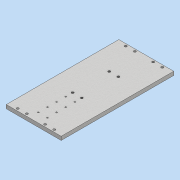
# Autodesk Inventor part: Wspornik pionowy osi Z
Saved by Autodesk Inventor 2018 (Build 220112000, 112)
## iProperties
Created: 2019-01-27
Part Number: Wspornik pionowy osi Z
Material: Ogólny
Document SubType Name: Modeling
Designer: Dawid
Density: 1 g/cm^3
Appearance: Aluminium odlewane
Author: Dawid
Autodesk Inventor part; units mm, degrees
ref_plane "YZ Plane" through (0, 0, 0) normal (1, 0, 0) x (0, 1, 0)
ref_plane "XZ Plane" through (0, 0, 0) normal (0, 1, 0) x (-1, 0, 0)
ref_plane "XY Plane" through (0, 0, 0) normal (0, 0, 1) x (1, 0, 0)
sketch "Szkic1" plane through (0, 0, 0) normal (0, 0, 1) x (1, 0, 0)
  line L0 (-50, -65) -> (50, -65)
  line L1 (50, -65) -> (50, 65)
  line L2 (50, 65) -> (-50, 65)
  line L3 (-50, 65) -> (-50, -65)
  line L4 (-50, -65) -> (50, 65) construction
  line L5 (50, -65) -> (-50, 65) construction
  point P0 (0, 0)
  dimension "d0" = 100
  dimension "d1" = 130
  constraints: 12 end point, 2 midpoint, 2 parallel, 1 horizontal, 1 perpendicular
  measures "d0" distance of L2.end L1.end
  measures "d1" distance of L1.end L0.end
extrude "Wyciągnięcie proste1" add sketch "Szkic1" along normal blind 8
sketch "Szkic2" plane through (0, 0, 8) normal (0, 0, 1) x (1, 0, 0)
  line L0 (-16.2, -31.5) -> (-16.2, -58.5)
  line L1 (-16.2, -58.5) -> (16.2, -58.5)
  line L2 (16.2, -31.5) -> (16.2, -58.5)
  line L3 (-16.2, -31.5) -> (16.2, -31.5)
  line L4 (-16.2, -58.5) -> (16.2, -58.5)
  line L5 (16.2, -31.5) -> (-16.2, -58.5)
  line L6 (16.2, -58.5) -> (-16.2, -31.5)
  line L7 (-10, -45) -> (-10, -53.5)
  line L8 (-8.5, -55) -> (8.5, -55)
  line L9 (10, -53.5) -> (10, -36.5)
  line L10 (8.5, -35) -> (-8.5, -35)
  line L11 (-10, -36.5) -> (-10, -45)
  circle A0 centre (10, -55) radius 1.5
  circle A1 centre (-10, -55) radius 1.5
  circle A2 centre (10, -35) radius 1.5
  circle A3 centre (-10, -35) radius 1.5
  line L12 (-50, -65) -> (50, -65) projected
  line L13 (-50, -65) -> (-50, -58.5)
  line L14 (-50, 65) -> (-50, -65) projected
  line L15 (-50, -58.5) -> (50, -58.5)
  line L16 (0, -58.5) -> (0, 0)
  line L17 (0, -45) -> (0, -58.5)
  point P0 (-16.2, -45)
  dimension "d4" = 3
  dimension "d5" = 3
  dimension "d6" = 3
  dimension "d7" = 3
  dimension "d8" = 6.5
  constraints: 32 end point, 8 point on circle, 4 centre point, 4 perpendicular, 3 midpoint, 1 parallel, 1 point on line, 1 vertical
  measures "d4" diameter of A0
  measures "d5" diameter of A1
  measures "d6" diameter of A2
  measures "d7" diameter of A3
  measures "d8" distance of L12.start L13.end
extrude "Wyciągnięcie proste2" cut sketch "Szkic2" against normal up to next contours A3 L6 | L6 A3 | A1 L5 | L5 A1 | A2 L5 | L5 A2 | A0 L6 | L6 A0
sketch "Szkic5" plane through (0, 0, 8) normal (0, 0, 1) x (1, 0, 0)
  line L0 (-16.2, 8.5) -> (-16.2, -18.5)
  line L1 (-16.2, -18.5) -> (16.2, -18.5)
  line L2 (16.2, 8.5) -> (16.2, -18.5)
  line L3 (-16.2, 8.5) -> (16.2, 8.5)
  line L4 (-16.2, -18.5) -> (16.2, -18.5)
  line L5 (16.2, 8.5) -> (-16.2, -18.5)
  line L6 (16.2, -18.5) -> (-16.2, 8.5)
  line L7 (-10, -5) -> (-10, -13.5)
  line L8 (-8.5, -15) -> (8.5, -15)
  line L9 (10, -13.5) -> (10, 3.5)
  line L10 (8.5, 5) -> (-8.5, 5)
  line L11 (-10, 3.5) -> (-10, -5)
  circle A0 centre (10, -15) radius 1.5
  circle A1 centre (-10, -15) radius 1.5
  circle A2 centre (10, 5) radius 1.5
  circle A3 centre (-10, 5) radius 1.5
  line L12 (-50, -65) -> (50, -65)
  line L13 (-50, -65) -> (-50, -58.5)
  line L14 (-50, 65) -> (-50, -65)
  line L15 (-50, -58.5) -> (50, -58.5)
  line L16 (0, -18.5) -> (0, 8.5)
  line L17 (0, -5) -> (0, -18.5)
  line L18 (0, 0) -> (0, -18.5)
  point P0 (-16.2, -5)
  dimension "d15" = 3
  dimension "d16" = 3
  dimension "d17" = 3
  dimension "d18" = 3
  dimension "d19" = 6.5
  dimension "d20" = 18.5
  constraints: 38 end point, 8 point on circle, 4 centre point, 4 perpendicular, 3 midpoint, 2 vertical, 1 parallel, 1 point on line
  measures "d15" diameter of A0
  measures "d16" diameter of A1
  measures "d17" diameter of A2
  measures "d18" diameter of A3
  measures "d19" distance of L12.start L13.end
  measures "d20" distance of L18.start L18.end
extrude "Wyciągnięcie proste5" cut sketch "Szkic5" against normal up to next contours A3 L6 | L6 A3 | A1 L5 | L5 A1 | A2 L5 | L5 A2 | A0 L6 | L6 A0
sketch "Szkic7" plane through (-50, 65, 0) normal (0, 1, 0) x (1, 0, 0)
  line L0 (100, 0) -> (0, 0) projected
  line L1 (0, 0) -> (0, -8) projected
  line L2 (100, -8) -> (0, -8) projected
  line L3 (100, 0) -> (100, -8) projected
  point P0 (50, 0)
extrude "Wyciągnięcie proste6" add sketch "Szkic7" along normal blind 45
sketch "Szkic8" plane through (0, 0, 0) normal (0, 0, -1) x (-1, 0, 0)
  line L0 (-20, 110) -> (-20, 10)
  line L1 (20, 10) -> (-20, 10)
  line L2 (20, 10) -> (20, 110)
  line L3 (-20, 110) -> (20, 110)
  line L4 (-20, 110) -> (20, 10)
  line L5 (20, 110) -> (-20, 10)
  line L6 (0, 0.7274) -> (0, 110)
  line L7 (0, 60) -> (0, 110)
  line L8 (0, 60) -> (0, 10)
  circle A0 centre (-10, 100) radius 2.5
  circle A1 centre (10, 100) radius 2.5
  circle A2 centre (-10, 20) radius 2.5
  circle A3 centre (10, 20) radius 2.5
  line L9 (-50, 110) -> (50, 110) projected
  line L10 (0, 110) -> (0, 109.7979)
  point P0 (0, 0)
  point P1 (-20, 60)
  dimension "d32" = 5
  dimension "d33" = 5
  dimension "d34" = 5
  dimension "d35" = 5
  constraints: 20 end point, 5 midpoint, 4 centre point, 2 vertical
  measures "d32" diameter of A0
  measures "d33" diameter of A1
  measures "d34" diameter of A2
  measures "d35" diameter of A3
extrude "Wyciągnięcie proste7" cut sketch "Szkic8" against normal up to next contours A0 | A1 | A2 | A3
thread "Gwint1" size "M5x0.8" class "6H" standard "ANSI Metric M Profile" full length
thread "Gwint2" size "M5x0.8" class "6H" standard "ANSI Metric M Profile" full length
thread "Gwint3" size "M5x0.8" class "6H" standard "ANSI Metric M Profile" full length
thread "Gwint4" size "M5x0.8" class "6H" standard "ANSI Metric M Profile" full length
sketch "Szkic9" plane through (0, 0, 0) normal (0, 0, -1) x (-1, 0, 0)
  circle A0 centre (-10, -15) radius 1.5 projected
  circle A1 centre (-10, 5) radius 1.5 projected
  circle A2 centre (10, -15) radius 1.5 projected
  circle A3 centre (10, 5) radius 1.5 projected
  circle A4 centre (-10, -55) radius 1.5 projected
  circle A5 centre (-10, -35) radius 1.5 projected
  circle A6 centre (10, -55) radius 1.5 projected
  circle A7 centre (10, -35) radius 1.5 projected
  line L0 (50, -65) -> (-50, -65) projected
  line L1 (50, -65) -> (50, 110) projected
  line L2 (-50, 110) -> (50, 110) projected
  line L3 (-50, -65) -> (-50, 110) projected
  point P0 (0, 0)
  constraints: 8 centre point
hole "Otwór2" at (10, 5, 0) at (-10, 5, 0) at (-10, -15, 0) at (10, -15, 0) at (10, -35, 0) at (-10, -35, 0) at (-10, -55, 0) at (10, -55, 0) direction (0, 0, 1) diameter 3 end through all countersink diameter 7 countersink angle 90
sketch "Szkic10" plane through (50, -65, 8) normal (1, 0, 0) x (0, 0, -1)
  line L0 (8, 0) -> (8, 175) projected
  line L1 (0, 175) -> (8, 175) projected
  line L2 (0, 0) -> (0, 175) projected
  line L3 (8, 0) -> (0, 0) projected
  point P0 (8, 65)
sketch "Szkic11" plane through (-50, -65, 0) normal (-1, 0, 0) x (0, 0, 1)
  line L0 (0, 0) -> (0, 175) projected
  line L1 (0, 0) -> (8, 0) projected
  line L2 (8, 0) -> (8, 175) projected
  line L3 (0, 175) -> (8, 175) projected
  point P0 (0, 65)
extrude "Wyciągnięcie proste8" add sketch "Szkic11" along normal blind 10
extrude "Wyciągnięcie proste9" add sketch "Szkic10" along normal blind 10
sketch "Szkic13" plane through (-60, -65, 0) normal (0, -1, 0) x (1, 0, 0)
  line L0 (0, 0) -> (120, 0) projected
  line L1 (120, 8) -> (120, 0) projected
  line L2 (120, 8) -> (0, 8) projected
  line L3 (0, 0) -> (0, 8) projected
  point P0 (60, 0)
extrude "Wyciągnięcie proste10" add sketch "Szkic13" along normal blind 10
sketch "Szkic14" plane through (0, 0, 8) normal (0, 0, 1) x (1, 0, 0)
  line L0 (60, -75) -> (-60, -75) projected
  line L1 (-60, 110) -> (-60, -75) projected
  line L2 (60, 110) -> (60, -75) projected
  line L3 (-60, -75) -> (-60, -65)
  line L4 (-60, 110) -> (-60, -75) projected
  line L5 (-60, -65) -> (60, -65)
  line L6 (-60, -65) -> (-60, -70)
  line L7 (-60, -70) -> (60, -70)
  line L8 (-60, -75) -> (-40, -75)
  line L9 (-60, -75) -> (60, -75) projected
  line L10 (-40, -75) -> (-40, -65)
  line L11 (-40, -75) -> (-20, -75)
  line L12 (-20, -75) -> (-20, -65)
  line L13 (-20, -75) -> (20, -75)
  line L14 (20, -75) -> (20, -65)
  line L15 (20, -75) -> (40, -75)
  line L16 (40, -75) -> (40, -65)
  circle A0 centre (-40, -70) radius 2.5
  circle A1 centre (-20, -70) radius 2.5
  circle A2 centre (20, -70) radius 2.5
  circle A3 centre (40, -70) radius 2.5
  point P0 (0, 0)
  dimension "d84" = 10
  dimension "d85" = 5
  dimension "d86" = 20
  dimension "d87" = 20
  dimension "d89" = 20
  dimension "d90" = 5
  dimension "d91" = 5
  dimension "d92" = 5
  dimension "d93" = 5
  dimension "d105" = 20
  constraints: 24 end point, 12 point on line, 6 perpendicular, 4 centre point, 4 midpoint
  measures "d84" distance of L0.end L3.end
  measures "d85" distance of L3.end L6.end
  measures "d86" distance of L0.end L8.end
  measures "d87" distance of L8.end L11.end
  measures "d89" distance of L13.end L15.end
  measures "d90" diameter of A0
  measures "d91" diameter of A1
  measures "d92" diameter of A2
  measures "d93" diameter of A3
  measures "d105" distance from line of L2 A3.centre
hole "Otwór5" at (-40, -70, 8) at (-20, -70, 8) at (20, -70, 8) at (40, -70, 8) direction (0, 0, -1) diameter 5 end through all
sketch "Szkic16" plane through (-50, 110, 0) normal (0, 1, 0) x (1, 0, 0)
  line L0 (-10, 0) -> (110, 0) projected
  line L1 (-10, -8) -> (-10, 0) projected
  line L2 (110, -8) -> (-10, -8) projected
  line L3 (110, 0) -> (110, -8) projected
  point P0 (50, 0)
extrude "Wyciągnięcie proste12" add sketch "Szkic16" along normal blind 61
sketch "Szkic17" plane through (0, 0, 0) normal (0, 0, -1) x (-1, 0, 0)
  line L0 (60, 161) -> (-60, 161)
  line L1 (-60, 346) -> (-60, 161)
  line L2 (60, 346) -> (60, 161)
  line L3 (-60, 161) -> (-60, 171)
  line L4 (-60, 346) -> (-60, 161)
  line L5 (-60, 171) -> (60, 171)
  line L6 (-60, 171) -> (-60, 166)
  line L7 (-60, 166) -> (60, 166)
  line L8 (-60, 161) -> (-40, 161)
  line L9 (-60, 161) -> (60, 161)
  line L10 (-40, 161) -> (-40, 171)
  line L11 (-40, 161) -> (-20, 161)
  line L12 (-20, 161) -> (-20, 171)
  line L13 (-20, 161) -> (20, 161)
  line L14 (20, 161) -> (20, 171)
  line L15 (20, 161) -> (40, 161)
  line L16 (40, 161) -> (40, 171)
  circle A0 centre (-40, 166) radius 2.5
  circle A1 centre (-20, 166) radius 2.5
  circle A2 centre (20, 166) radius 2.5
  circle A3 centre (40, 166) radius 2.5
  line L17 (-60, 171) -> (60, 171) projected
  point P0 (0, 0)
  point P1 (0, 236)
  dimension "d106" = 10
  dimension "d107" = 5
  dimension "d108" = 20
  dimension "d109" = 20
  dimension "d110" = 20
  dimension "d111" = 5
  dimension "d112" = 5
  dimension "d113" = 5
  dimension "d114" = 5
  dimension "d115" = 20
  constraints: 34 end point, 12 point on line, 6 perpendicular, 4 centre point, 4 midpoint
  measures "d106" distance of L0.end L3.end
  measures "d107" distance of L3.end L6.end
  measures "d108" distance of L0.end L8.end
  measures "d109" distance of L8.end L11.end
  measures "d110" distance of L13.end L15.end
  measures "d111" diameter of A0
  measures "d112" diameter of A1
  measures "d113" diameter of A2
  measures "d114" diameter of A3
  measures "d115" distance from line of L2 A3.centre
extrude "Wyciągnięcie proste13" cut sketch "Szkic17" against normal up to next contours A3 L7 L16 | L16 L7 A3 | L7 L16 A3 | A2 L7 L14 | L14 L7 A2 | L7 A3 L16 | A1 L7 L12 | L12 L7 A1 | L14 A2 L7 | L7 A2 L14 | A0 L7 L10 | L10 L7 A0 | L12 A1 L7 | L7 A1 L12 | L10 A0 L7 | L7 A0 L10
